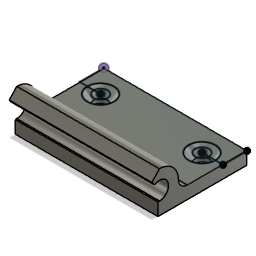
Thomas_TT_cover_hinge (Autodesk Fusion 360 design; units mm, degrees)
Autodesk Fusion 360 part; units mm, degrees
note: some values were not read from the file. Set by a fixed rule: which sketch regions a step uses.
sketch "Sketch1" plane through (0, 0, 0) normal (0, 1, 0) x (1, 0, 0)
  line L0 (0, 0) -> (47.6, 0)
  line L1 (47.6, 0) -> (47.6, -29.5)
  line L2 (47.6, -29.5) -> (0, -29.5)
  line L3 (0, -29.5) -> (0, 0)
  dimension "d1" = 47.6
  dimension "d2" = 29.5
  constraint horizontal L0
  constraint vertical L1
  constraint horizontal L2
  constraint vertical L3
  constraint coincident L0.start L3.end
  measures "d1" distance of L0.start L0.end
  measures "d2" distance of L0.start L2.end
extrude "Extrude1" add sketch "Sketch1" along normal blind 4.2
sketch "Sketch2" plane through (47.6, 0, 0) normal (1, 0, 0) x (0, 0, -1)
  line L0 (-29.5, 0) -> (0, 0)
  line L1 (0, 0) -> (0, 4.2)
  line L2 (0, 4.2) -> (-29.5, 4.2)
  line L3 (-29.5, 4.2) -> (-29.5, 0)
  line L4 (-29.5, 4.2) -> (-29, 4.2)
  line L5 (-29, 4.2) -> (-29, 7.2)
  circle A0 centre (-29, 7.2) radius 3
  circle A1 centre (-29, 7.2) radius 6.3
  line L6 (-29, 7.2) -> (-29, 13.5)
  line L7 (-26, 7.2) -> (-26, 12.7399)
  line L8 (-26, 12.7399) -> (-31.5, 12.7399)
  line L9 (-31.5, 12.7399) -> (-31.5, 8.8583)
  line L10 (-31.5, 10.7991) -> (-29, 13.5)
  line L11 (-31.5, 10.7991) -> (-30.6784, 9.6865)
  dimension "d5" = 0.5
  dimension "d6" = 3
  dimension "d7" = 6
  dimension "d8" = 3.3
  dimension "d9" = 5.5
  constraint coincident L2.end L3.start
  constraint perpendicular L3 L4
  constraint perpendicular L4 L5
  constraint coincident L5.end A0.centre
  constraint coincident A1 L6.end
  constraint parallel L5 L6
  constraint coincident A0 L7.start
  constraint coincident A1 L7.end
  constraint tangent A0 L7
  constraint parallel L6 L7
  constraint perpendicular L7 L8
  constraint coincident A0 L9.end
  constraint perpendicular L8 L9
  constraint midpoint L9 L10.start
  constraint coincident A0 L11.end
  measures "d5" distance of L2.end L4.end
  measures "d6" distance of L4.end L5.end
  measures "d7" diameter of A0
  measures "d9" distance of L7.end L8.end
extrude "Extrude2" add sketch "Sketch2" against normal blind 48 contours A1 L6 L8 | L6 L8 L10 | L2 A0 A1 L7 | A0 L6 L7 L8 | A0 L6 L8 L10 L11
extrude "Extrude3" cut 1 faces at (-0.4, 11.4891, 29.9783) along direction (1, 0, 0) blind 0.4
fillet "Fillet1" radius 0.25 1 edges at (23.8, 9.6865, 30.6784)
fillet "Fillet2" radius 3 1 edges at (23.8, 4.2, 23.4601)
sketch "Sketch3" plane through (0, 4.2, 0) normal (0, 1, 0) x (-1, 0, 0)
  line L0 (0, 19.7) -> (-47.6, 19.7)
  line L1 (-47.6, 19.7) -> (-47.6, 0)
  line L2 (-47.6, 0) -> (0, 0)
  line L3 (0, 0) -> (0, 19.7)
  line L4 (0, 0) -> (0, 8)
  line L5 (0, 8) -> (-6.95, 8)
  circle A0 centre (-6.95, 8) radius 2.25
  line L6 (-47.6, 0) -> (-47.6, 8)
  line L7 (-47.6, 8) -> (-40.65, 8)
  circle A1 centre (-40.65, 8) radius 2.25
  circle A2 centre (-6.95, 8) radius 4.4
  circle A3 centre (-40.65, 8) radius 4.4
  dimension "d18" = 8
  dimension "d19" = 6.95
  dimension "d20" = 4.5
  dimension "d21" = 8
  dimension "d22" = 6.95
  dimension "d23" = 4.5
  dimension "d24" = 8.8
  dimension "d25" = 8.8
  constraint coincident L2.end L3.start
  constraint perpendicular L2 L4
  constraint perpendicular L4 L5
  constraint coincident L5.end A0.centre
  constraint coincident L1.end L2.start
  constraint coincident L1 L6.end
  constraint perpendicular L6 L7
  constraint coincident L7.end A1.centre
  constraint concentric A0 A2
  constraint concentric A1 A3
  measures "d18" distance of L2.end L4.end
  measures "d19" distance of L4.end L5.end
  measures "d20" diameter of A0
  measures "d21" distance of L1.end L6.end
  measures "d22" distance of L6.end L7.end
  measures "d23" diameter of A1
  measures "d24" diameter of A2
  measures "d25" diameter of A3
extrude "Extrude4" cut sketch "Sketch3" against normal blind 6 contours A1
extrude "Extrude5" cut sketch "Sketch3" against normal blind 9 contours A0
ref_plane "WorkPlane1" through (23.8, 1.4, 9.85) normal (0, 1, 0) x (-1, 0, 0)
sketch "Sketch4" plane through (0, 1.4, 0) normal (0, 1, 0) x (1, 0, 0)
  circle A0 centre (6.95, -8) radius 2.25
  circle A1 centre (40.65, -8) radius 2.25
  point P0 (6.95, -8)
loft "Loft1" cut profiles "Sketch4", "Sketch3" section 1 contours A0 section 2 contours A2
loft "Loft2" cut profiles "Sketch4", "Sketch3" section 1 contours A1 section 2 contours A3
extrude "Extrude6" cut 1 faces at (47.6, 1.4, 16.4) along direction (-1, 0, 0) blind 0.1
extrude "Extrude7" cut 1 faces at (0, 1.4, 16.4) along direction (1, 0, 0) blind 0.1
equation "d19 = 4.7 mm + ( ( 4.5 / 2 ) * 1 mm )"
named bodies: "hinge"
